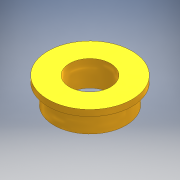
# Autodesk Inventor part: ベアリング　内径4
Saved by Autodesk Inventor 2020.2 (Build 242310000, 310)
## iProperties
Created: 2018-03-28
Part Number: ベアリング　内径4
Material: 一般
Document SubType Name: Modeling
Designer: Takumi
Mass: 0.35 g
Surface Area: 1.69143 cm^2
Volume: 0.0733907 cm^3
Density: 4.76899 g/cm^3
Appearance: 溶接 - 真鍮
Author: Takumi
Autodesk Inventor part; units mm, degrees
ref_plane "YZ Plane" through (0, 0, 0) normal (1, 0, 0) x (0, 1, 0)
ref_plane "XZ Plane" through (0, 0, 0) normal (0, 1, 0) x (-1, 0, 0)
ref_plane "XY Plane" through (0, 0, 0) normal (0, 0, 1) x (1, 0, 0)
sketch "スケッチ1" plane through (0, 0, 0) normal (0, 0, 1) x (1, 0, 0)
  circle A0 centre (0, 0) radius 2
  circle A1 centre (0, 0) radius 3.5
  circle A2 centre (0, 0) radius 4.1
  dimension "d0" = 4
  dimension "d1" = 7
  dimension "d2" = 8.2
  constraints: 3 centre point, 3 coincident
  measures "d0" diameter of A0
  measures "d1" diameter of A1
  measures "d2" diameter of A2
extrude "押し出し1" add sketch "スケッチ1" along normal blind 0.6 contours A1 | A2
extrude "押し出し2" add sketch "スケッチ1" against normal blind 1.9 contours A1
